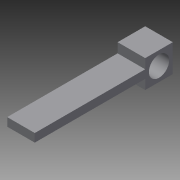
# Autodesk Inventor part: 000207
Saved by Autodesk Inventor 2015 (Build 190159000, 159)
## iProperties
Created: 2015-05-27
Part Number: 000207
Material: Generic
Document SubType Name: Modeling
Designer: Wesley
Density: 1 g/cm^3
Appearance: Default
Author: Wesley
Autodesk Inventor part; units mm, degrees
ref_plane "YZ Plane" through (0, 0, 0) normal (1, 0, 0) x (0, 1, 0)
ref_plane "XZ Plane" through (0, 0, 0) normal (0, 1, 0) x (-1, 0, 0)
ref_plane "XY Plane" through (0, 0, 0) normal (0, 0, 1) x (1, 0, 0)
sketch "Sketch1" plane through (0, 0, 0) normal (0, 0, 1) x (1, 0, 0)
  line L0 (0, 0) -> (6.35, 0)
  line L1 (6.35, 0) -> (6.35, 1.905)
  line L2 (6.35, 1.905) -> (0, 1.905)
  line L3 (0, 1.905) -> (0, 0)
  dimension "d0" = 1.905
  dimension "d1" = 6.35
  constraints: 8 end point, 2 parallel, 1 horizontal, 1 perpendicular
  measures "d0" distance of L2.end L0.start
  measures "d1" distance of L0.start L0.end
extrude "Extrusion1" add sketch "Sketch1" along normal blind 31.75
sketch "Sketch2" plane through (0, 1.905, 0) normal (0, 1, 0) x (1, 0, 0)
  line L0 (6.35, 0) -> (6.35, -31.75) projected
  line L1 (0, 0) -> (6.35, 0)
  line L2 (6.35, 0) -> (6.35, -6.35)
  line L3 (6.35, -6.35) -> (0, -6.35)
  line L4 (0, -6.35) -> (0, 0)
  dimension "d4" = 6.35
  constraints: 8 end point, 2 parallel, 1 horizontal, 1 perpendicular, 1 point on line
  measures "d4" distance of L1.end L2.end
extrude "Extrusion2" add sketch "Sketch2" along normal blind 2.2225 and the other way blind 4.1275
sketch "Sketch3" plane through (6.35, 0, 31.75) normal (1, 0, 0) x (0, 0, -1)
  line L0 (21.2753, 0.9525) -> (48.2824, 0.9525) construction
  line L1 (28.575, 14.3554) -> (28.575, -13.5982) construction
  line L2 (31.75, 4.1275) -> (31.75, -2.2225) construction
  line L3 (25.4, 4.1275) -> (31.75, 4.1275) construction
  line L4 (31.75, -2.2225) -> (25.4, -2.2225) construction
  circle A0 centre (28.575, 0.9525) radius 2.3343
  point P0 (31.75, 0)
  dimension "d9" = 3.175
  dimension "d11" = 3.175
  dimension "d12" = 4.6685
  constraints: 4 end point, 2 point on line, 1 centre point, 1 horizontal, 1 vertical
  measures "d9" distance between parallel lines of L2 L1
  measures "d11" distance between parallel lines of L0 L4
  measures "d12" diameter of A0
extrude "Extrusion3" cut sketch "Sketch3" against normal through all
body "Solid1"
